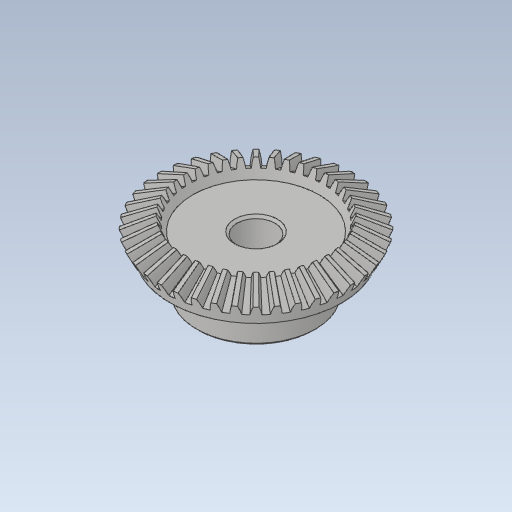
# Autodesk Inventor part: PB1-4020_On
Saved by Autodesk Inventor 2024 (Build 280153000, 153)
## iProperties
Created: 2023-09-03
Part Number: PB1-4020_On
Material: Generic
Catalog Web Link: www.cadenas.de
Description: Plastic Bevel Gears (PB)-R-
Vendor: KHK
Document SubType Name: Modeling
Designer: psAdmin
Manufacturer: KHK
Mass: 8.42838 g
Surface Area: 44.7487 cm^2
Volume: 8.42838 cm^3
Density: 1 g/cm^3
Appearance: PSOLRGB-175-175-175
Category: PARTsolutions
Company: KHK
PSOL_IDENT_0: {$CADENAS_DATA/23d-libs/khk/bevel_gears/pb_r.prj},185 {VTYP=3D},{NB=PB1-4020_On},{LINA=PB1-4020},{NN=
PSOL_IDENT_1: Plastic Bevel Gears (PB)-R},{DATE=06.10.2022 23:14:38},{GEOMDATE=20.03.2019 11:32:20},{VERSION=},{LI
PSOL_IDENT_2: NEID=340},{WBVAR=TOOTH},{WBNUMERIC=}  {NB=PB1-4020_On},{LINA=PB1-4020},{KT=DUMMY},{CN=PB1-4020},{M=1
PSOL_IDENT_3: .0},{Z=40},{A=8},{B=25},{C=40.0},{D=40.59},{E=22},{F=15.07},{G=12.59},{H=8.00},{I=12.0},{J=6},{K=26.
PSOL_IDENT_4: 58},{L=65.60},{S=B4},{PN=PB1-2040},{WMF=B4005.WMF},{X=0.5},{Y=0.5},{R=1.0},{H1=36.00},{VERS=5},{TOOT
PSOL_IDENT_5: H=On},{ANGLE=28.000}
NB: PB1-4020_On
NN: Plastic Bevel Gears (PB)-R
NBSYN: $CN._$TOOTH.
LINA: PB1-4020
CATALOG: KHK
CN: PB1-4020
M: 1
Z: 40
A: 8
B: 25
C: 40
D: 40.59
E: 22
F: 15.07
G: 12.59
H: 8
I: 12
J: 6
K: 26.58
L: 65.6
S: B4
PN: PB1-2040
WMF: B4005.WMF
X: 0.5
Y: 0.5
R: 1
H1: 36
VERS: 5
TOOTH: On
ANGLE: 28
SUPPLIER: KHK
ARTICLENO: PB1-4020_On
BOMINFO: PB1-4020
CREATOR: CADENAS GmbH
Title: PB1-4020
Author: Cadenas PARTsolutions
Autodesk Inventor part; units mm, degrees
sketch "Sketch_5" plane through (0, -14, 0) normal (0, 1, 0) x (1, 0, 0)
  arc A0 (-0.3975, 31.6288) -> (-0.999, 21.1842) centre (59.8613, 22.9187) ccw
  arc A1 (-0.999, 21.1842) -> (-2.3272, 21.0797) centre (0, 0) ccw
  arc A2 (-2.3272, 21.0797) -> (-4.5552, 31.3016) centre (-62.7095, 13.2721) ccw
  arc A3 (-4.5552, 31.3016) -> (-5.3404, 31.1772) centre (0, 0) ccw
  arc A4 (-5.3404, 31.1772) -> (-4.3007, 20.7671) centre (55.539, 32.0009) ccw
  arc A5 (-4.3007, 20.7671) -> (-5.5961, 20.4561) centre (0, 0) ccw
  arc A6 (-5.5961, 20.4561) -> (-9.3958, 30.2036) centre (-64.0137, 3.2988) ccw
  arc A7 (-9.3958, 30.2036) -> (-10.1519, 29.9579) centre (0, 0) ccw
  arc A8 (-10.1519, 29.9579) -> (-7.4964, 19.8387) centre (49.8492, 40.2951) ccw
  arc A9 (-7.4964, 19.8387) -> (-8.7273, 19.3288) centre (0, 0) ccw
  arc A10 (-8.7273, 19.3288) -> (-14.005, 28.3619) centre (-63.7416, -6.7558) ccw
  arc A11 (-14.005, 28.3619) -> (-14.7133, 28.001) centre (0, 0) ccw
  arc A12 (-14.7133, 28.001) -> (-10.5076, 18.4217) centre (42.9319, 47.5971) ccw
  arc A13 (-10.5076, 18.4217) -> (-11.6435, 17.7256) centre (0, 0) ccw
  arc A14 (-11.6435, 17.7256) -> (-18.2694, 25.8219) centre (-61.9, -16.644) ccw
  arc A15 (-18.2694, 25.8219) -> (-18.9125, 25.3546) centre (0, 0) ccw
  arc A16 (-18.9125, 25.3546) -> (-13.26, 16.5512) centre (34.9575, 53.7272) ccw
  arc A17 (-13.26, 16.5512) -> (-14.2731, 15.6859) centre (0, 0) ccw
  arc A18 (-14.2731, 15.6859) -> (-22.0839, 22.646) centre (-58.5343, -26.1224) ccw
  arc A19 (-22.0839, 22.646) -> (-22.646, 22.0839) centre (0, 0) ccw
  arc A20 (-22.646, 22.0839) -> (-15.6859, 14.2731) centre (26.1224, 58.5343) ccw
  arc A21 (-15.6859, 14.2731) -> (-16.5512, 13.26) centre (0, 0) ccw
  arc A22 (-16.5512, 13.26) -> (-25.3546, 18.9125) centre (-53.7272, -34.9575) ccw
  arc A23 (-25.3546, 18.9125) -> (-25.8219, 18.2694) centre (0, 0) ccw
  arc A24 (-25.8219, 18.2694) -> (-17.7256, 11.6435) centre (16.644, 61.9) ccw
  arc A25 (-17.7256, 11.6435) -> (-18.4217, 10.5076) centre (0, 0) ccw
  arc A26 (-18.4217, 10.5076) -> (-28.001, 14.7133) centre (-47.5971, -42.9319) ccw
  arc A27 (-28.001, 14.7133) -> (-28.3619, 14.005) centre (0, 0) ccw
  arc A28 (-28.3619, 14.005) -> (-19.3288, 8.7273) centre (6.7558, 63.7416) ccw
  arc A29 (-19.3288, 8.7273) -> (-19.8387, 7.4964) centre (0, 0) ccw
  arc A30 (-19.8387, 7.4964) -> (-29.9579, 10.1519) centre (-40.2951, -49.8492) ccw
  arc A31 (-29.9579, 10.1519) -> (-30.2036, 9.3958) centre (0, 0) ccw
  arc A32 (-30.2036, 9.3958) -> (-20.4561, 5.5961) centre (-3.2988, 64.0137) ccw
  arc A33 (-20.4561, 5.5961) -> (-20.7671, 4.3007) centre (0, 0) ccw
  arc A34 (-20.7671, 4.3007) -> (-31.1772, 5.3404) centre (-32.0009, -55.539) ccw
  arc A35 (-31.1772, 5.3404) -> (-31.3016, 4.5552) centre (0, 0) ccw
  arc A36 (-31.3016, 4.5552) -> (-21.0797, 2.3272) centre (-13.2721, 62.7095) ccw
  arc A37 (-21.0797, 2.3272) -> (-21.1842, 0.999) centre (0, 0) ccw
  arc A38 (-21.1842, 0.999) -> (-31.6288, 0.3975) centre (-22.9187, -59.8613) ccw
  arc A39 (-31.6288, 0.3975) -> (-31.6288, -0.3975) centre (0, 0) ccw
  arc A40 (-31.6288, -0.3975) -> (-21.1842, -0.999) centre (-22.9187, 59.8613) ccw
  arc A41 (-21.1842, -0.999) -> (-21.0797, -2.3272) centre (0, 0) ccw
  arc A42 (-21.0797, -2.3272) -> (-31.3016, -4.5552) centre (-13.2721, -62.7095) ccw
  arc A43 (-31.3016, -4.5552) -> (-31.1772, -5.3404) centre (0, 0) ccw
  arc A44 (-31.1772, -5.3404) -> (-20.7671, -4.3007) centre (-32.0009, 55.539) ccw
  arc A45 (-20.7671, -4.3007) -> (-20.4561, -5.5961) centre (0, 0) ccw
  arc A46 (-20.4561, -5.5961) -> (-30.2036, -9.3958) centre (-3.2988, -64.0137) ccw
  arc A47 (-30.2036, -9.3958) -> (-29.9579, -10.1519) centre (0, 0) ccw
  arc A48 (-29.9579, -10.1519) -> (-19.8387, -7.4964) centre (-40.2951, 49.8492) ccw
  arc A49 (-19.8387, -7.4964) -> (-19.3288, -8.7273) centre (0, 0) ccw
  arc A50 (-19.3288, -8.7273) -> (-28.3619, -14.005) centre (6.7558, -63.7416) ccw
  arc A51 (-28.3619, -14.005) -> (-28.001, -14.7133) centre (0, 0) ccw
  arc A52 (-28.001, -14.7133) -> (-18.4217, -10.5076) centre (-47.5971, 42.9319) ccw
  arc A53 (-18.4217, -10.5076) -> (-17.7256, -11.6435) centre (0, 0) ccw
  arc A54 (-17.7256, -11.6435) -> (-25.8219, -18.2694) centre (16.644, -61.9) ccw
  arc A55 (-25.8219, -18.2694) -> (-25.3546, -18.9125) centre (0, 0) ccw
  arc A56 (-25.3546, -18.9125) -> (-16.5512, -13.26) centre (-53.7272, 34.9575) ccw
  arc A57 (-16.5512, -13.26) -> (-15.6859, -14.2731) centre (0, 0) ccw
  arc A58 (-15.6859, -14.2731) -> (-22.646, -22.0839) centre (26.1224, -58.5343) ccw
  arc A59 (-22.646, -22.0839) -> (-22.0839, -22.646) centre (0, 0) ccw
  arc A60 (-22.0839, -22.646) -> (-14.2731, -15.6859) centre (-58.5343, 26.1224) ccw
  arc A61 (-14.2731, -15.6859) -> (-13.26, -16.5512) centre (0, 0) ccw
  arc A62 (-13.26, -16.5512) -> (-18.9125, -25.3546) centre (34.9575, -53.7272) ccw
  arc A63 (-18.9125, -25.3546) -> (-18.2694, -25.8219) centre (0, 0) ccw
  arc A64 (-18.2694, -25.8219) -> (-11.6435, -17.7256) centre (-61.9, 16.644) ccw
  arc A65 (-11.6435, -17.7256) -> (-10.5076, -18.4217) centre (0, 0) ccw
  arc A66 (-10.5076, -18.4217) -> (-14.7133, -28.001) centre (42.9319, -47.5971) ccw
  arc A67 (-14.7133, -28.001) -> (-14.005, -28.3619) centre (0, 0) ccw
  arc A68 (-14.005, -28.3619) -> (-8.7273, -19.3288) centre (-63.7416, 6.7558) ccw
  arc A69 (-8.7273, -19.3288) -> (-7.4964, -19.8387) centre (0, 0) ccw
  arc A70 (-7.4964, -19.8387) -> (-10.1519, -29.9579) centre (49.8492, -40.2951) ccw
  arc A71 (-10.1519, -29.9579) -> (-9.3958, -30.2036) centre (0, 0) ccw
  arc A72 (-9.3958, -30.2036) -> (-5.5961, -20.4561) centre (-64.0137, -3.2988) ccw
  arc A73 (-5.5961, -20.4561) -> (-4.3007, -20.7671) centre (0, 0) ccw
  arc A74 (-4.3007, -20.7671) -> (-5.3404, -31.1772) centre (55.539, -32.0009) ccw
  arc A75 (-5.3404, -31.1772) -> (-4.5552, -31.3016) centre (0, 0) ccw
  arc A76 (-4.5552, -31.3016) -> (-2.3272, -21.0797) centre (-62.7095, -13.2721) ccw
  arc A77 (-2.3272, -21.0797) -> (-0.999, -21.1842) centre (0, 0) ccw
  arc A78 (-0.999, -21.1842) -> (-0.3975, -31.6288) centre (59.8613, -22.9187) ccw
  arc A79 (-0.3975, -31.6288) -> (0.3975, -31.6288) centre (0, 0) ccw
  arc A80 (0.3975, -31.6288) -> (0.999, -21.1842) centre (-59.8613, -22.9187) ccw
  arc A81 (0.999, -21.1842) -> (2.3272, -21.0797) centre (0, 0) ccw
  arc A82 (2.3272, -21.0797) -> (4.5552, -31.3016) centre (62.7095, -13.2721) ccw
  arc A83 (4.5552, -31.3016) -> (5.3404, -31.1772) centre (0, 0) ccw
  arc A84 (5.3404, -31.1772) -> (4.3007, -20.7671) centre (-55.539, -32.0009) ccw
  arc A85 (4.3007, -20.7671) -> (5.5961, -20.4561) centre (0, 0) ccw
  arc A86 (5.5961, -20.4561) -> (9.3958, -30.2036) centre (64.0137, -3.2988) ccw
  arc A87 (9.3958, -30.2036) -> (10.1519, -29.9579) centre (0, 0) ccw
  arc A88 (10.1519, -29.9579) -> (7.4964, -19.8387) centre (-49.8492, -40.2951) ccw
  arc A89 (7.4964, -19.8387) -> (8.7273, -19.3288) centre (0, 0) ccw
  arc A90 (8.7273, -19.3288) -> (14.005, -28.3619) centre (63.7416, 6.7558) ccw
  arc A91 (14.005, -28.3619) -> (14.7133, -28.001) centre (0, 0) ccw
  arc A92 (14.7133, -28.001) -> (10.5076, -18.4217) centre (-42.9319, -47.5971) ccw
  arc A93 (10.5076, -18.4217) -> (11.6435, -17.7256) centre (0, 0) ccw
  arc A94 (11.6435, -17.7256) -> (18.2694, -25.8219) centre (61.9, 16.644) ccw
  arc A95 (18.2694, -25.8219) -> (18.9125, -25.3546) centre (0, 0) ccw
  arc A96 (18.9125, -25.3546) -> (13.26, -16.5512) centre (-34.9575, -53.7272) ccw
  arc A97 (13.26, -16.5512) -> (14.2731, -15.6859) centre (0, 0) ccw
  arc A98 (14.2731, -15.6859) -> (22.0839, -22.646) centre (58.5343, 26.1224) ccw
  arc A99 (22.0839, -22.646) -> (22.646, -22.0839) centre (0, 0) ccw
  arc A100 (22.646, -22.0839) -> (15.6859, -14.2731) centre (-26.1224, -58.5343) ccw
  arc A101 (15.6859, -14.2731) -> (16.5512, -13.26) centre (0, 0) ccw
  arc A102 (16.5512, -13.26) -> (25.3546, -18.9125) centre (53.7272, 34.9575) ccw
  arc A103 (25.3546, -18.9125) -> (25.8219, -18.2694) centre (0, 0) ccw
  arc A104 (25.8219, -18.2694) -> (17.7256, -11.6435) centre (-16.644, -61.9) ccw
  arc A105 (17.7256, -11.6435) -> (18.4217, -10.5076) centre (0, 0) ccw
  arc A106 (18.4217, -10.5076) -> (28.001, -14.7133) centre (47.5971, 42.9319) ccw
  arc A107 (28.001, -14.7133) -> (28.3619, -14.005) centre (0, 0) ccw
  arc A108 (28.3619, -14.005) -> (19.3288, -8.7273) centre (-6.7558, -63.7416) ccw
  arc A109 (19.3288, -8.7273) -> (19.8387, -7.4964) centre (0, 0) ccw
  arc A110 (19.8387, -7.4964) -> (29.9579, -10.1519) centre (40.2951, 49.8492) ccw
  arc A111 (29.9579, -10.1519) -> (30.2036, -9.3958) centre (0, 0) ccw
  arc A112 (30.2036, -9.3958) -> (20.4561, -5.5961) centre (3.2988, -64.0137) ccw
  arc A113 (20.4561, -5.5961) -> (20.7671, -4.3007) centre (0, 0) ccw
  arc A114 (20.7671, -4.3007) -> (31.1772, -5.3404) centre (32.0009, 55.539) ccw
  arc A115 (31.1772, -5.3404) -> (31.3016, -4.5552) centre (0, 0) ccw
  arc A116 (31.3016, -4.5552) -> (21.0797, -2.3272) centre (13.2721, -62.7095) ccw
  arc A117 (21.0797, -2.3272) -> (21.1842, -0.999) centre (0, 0) ccw
  arc A118 (21.1842, -0.999) -> (31.6288, -0.3975) centre (22.9187, 59.8613) ccw
  arc A119 (31.6288, -0.3975) -> (31.6288, 0.3975) centre (0, 0) ccw
  arc A120 (31.6288, 0.3975) -> (21.1842, 0.999) centre (22.9187, -59.8613) ccw
  arc A121 (21.1842, 0.999) -> (21.0797, 2.3272) centre (0, 0) ccw
  arc A122 (21.0797, 2.3272) -> (31.3016, 4.5552) centre (13.2721, 62.7095) ccw
  arc A123 (31.3016, 4.5552) -> (31.1772, 5.3404) centre (0, 0) ccw
  arc A124 (31.1772, 5.3404) -> (20.7671, 4.3007) centre (32.0009, -55.539) ccw
  arc A125 (20.7671, 4.3007) -> (20.4561, 5.5961) centre (0, 0) ccw
  arc A126 (20.4561, 5.5961) -> (30.2036, 9.3958) centre (3.2988, 64.0137) ccw
  arc A127 (30.2036, 9.3958) -> (29.9579, 10.1519) centre (0, 0) ccw
  arc A128 (29.9579, 10.1519) -> (19.8387, 7.4964) centre (40.2951, -49.8492) ccw
  arc A129 (19.8387, 7.4964) -> (19.3288, 8.7273) centre (0, 0) ccw
  arc A130 (19.3288, 8.7273) -> (28.3619, 14.005) centre (-6.7558, 63.7416) ccw
  arc A131 (28.3619, 14.005) -> (28.001, 14.7133) centre (0, 0) ccw
  arc A132 (28.001, 14.7133) -> (18.4217, 10.5076) centre (47.5971, -42.9319) ccw
  arc A133 (18.4217, 10.5076) -> (17.7256, 11.6435) centre (0, 0) ccw
  arc A134 (17.7256, 11.6435) -> (25.8219, 18.2694) centre (-16.644, 61.9) ccw
  arc A135 (25.8219, 18.2694) -> (25.3546, 18.9125) centre (0, 0) ccw
  arc A136 (25.3546, 18.9125) -> (16.5512, 13.26) centre (53.7272, -34.9575) ccw
  arc A137 (16.5512, 13.26) -> (15.6859, 14.2731) centre (0, 0) ccw
  arc A138 (15.6859, 14.2731) -> (22.646, 22.0839) centre (-26.1224, 58.5343) ccw
  arc A139 (22.646, 22.0839) -> (22.0839, 22.646) centre (0, 0) ccw
  arc A140 (22.0839, 22.646) -> (14.2731, 15.6859) centre (58.5343, -26.1224) ccw
  arc A141 (14.2731, 15.6859) -> (13.26, 16.5512) centre (0, 0) ccw
  arc A142 (13.26, 16.5512) -> (18.9125, 25.3546) centre (-34.9575, 53.7272) ccw
  arc A143 (18.9125, 25.3546) -> (18.2694, 25.8219) centre (0, 0) ccw
  arc A144 (18.2694, 25.8219) -> (11.6435, 17.7256) centre (61.9, -16.644) ccw
  arc A145 (11.6435, 17.7256) -> (10.5076, 18.4217) centre (0, 0) ccw
  arc A146 (10.5076, 18.4217) -> (14.7133, 28.001) centre (-42.9319, 47.5971) ccw
  arc A147 (14.7133, 28.001) -> (14.005, 28.3619) centre (0, 0) ccw
  arc A148 (14.005, 28.3619) -> (8.7273, 19.3288) centre (63.7416, -6.7558) ccw
  arc A149 (8.7273, 19.3288) -> (7.4964, 19.8387) centre (0, 0) ccw
  arc A150 (7.4964, 19.8387) -> (10.1519, 29.9579) centre (-49.8492, 40.2951) ccw
  arc A151 (10.1519, 29.9579) -> (9.3958, 30.2036) centre (0, 0) ccw
  arc A152 (9.3958, 30.2036) -> (5.5961, 20.4561) centre (64.0137, 3.2988) ccw
  arc A153 (5.5961, 20.4561) -> (4.3007, 20.7671) centre (0, 0) ccw
  arc A154 (4.3007, 20.7671) -> (5.3404, 31.1772) centre (-55.539, 32.0009) ccw
  arc A155 (5.3404, 31.1772) -> (4.5552, 31.3016) centre (0, 0) ccw
  arc A156 (4.5552, 31.3016) -> (2.3272, 21.0797) centre (62.7095, 13.2721) ccw
  arc A157 (2.3272, 21.0797) -> (0.999, 21.1842) centre (0, 0) ccw
  arc A158 (0.999, 21.1842) -> (0.3975, 31.6288) centre (-59.8613, 22.9187) ccw
  arc A159 (0.3975, 31.6288) -> (-0.3975, 31.6288) centre (0, 0) ccw
  constraints: 320 point on circle, 160 centre point
sketch "Sketch_6" plane through (0, -6.93, 0) normal (0, 1, 0) x (1, 0, 0)
  arc A0 (-0.2948, 15.6369) -> (-0.61, 9.6964) centre (39.9716, 10.5213) ccw
  arc A1 (-0.61, 9.6964) -> (-0.9143, 9.6725) centre (0, 0) ccw
  arc A2 (-0.9143, 9.6725) -> (-2.155, 15.4905) centre (-41.1254, 4.1389) ccw
  arc A3 (-2.155, 15.4905) -> (-2.7373, 15.3983) centre (0, 0) ccw
  arc A4 (-2.7373, 15.3983) -> (-2.1194, 9.4816) centre (37.8336, 16.6447) ccw
  arc A5 (-2.1194, 9.4816) -> (-2.4162, 9.4104) centre (0, 0) ccw
  arc A6 (-2.4162, 9.4104) -> (-4.5517, 14.9627) centre (-41.2665, -2.3455) ccw
  arc A7 (-4.5517, 14.9627) -> (-5.1124, 14.7805) centre (0, 0) ccw
  arc A8 (-5.1124, 14.7805) -> (-3.5766, 9.0334) centre (34.764, 22.3583) ccw
  arc A9 (-3.5766, 9.0334) -> (-3.8585, 8.9166) centre (0, 0) ccw
  arc A10 (-3.8585, 8.9166) -> (-6.8363, 14.0664) centre (-40.3915, -8.7721) ccw
  arc A11 (-6.8363, 14.0664) -> (-7.3617, 13.7987) centre (0, 0) ccw
  arc A12 (-7.3617, 13.7987) -> (-4.9457, 8.3626) centre (30.8383, 27.5213) ccw
  arc A13 (-4.9457, 8.3626) -> (-5.2059, 8.2032) centre (0, 0) ccw
  arc A14 (-5.2059, 8.2032) -> (-8.9526, 12.8238) centre (-38.522, -14.9828) ccw
  arc A15 (-8.9526, 12.8238) -> (-9.4296, 12.4772) centre (0, 0) ccw
  arc A16 (-9.4296, 12.4772) -> (-6.193, 7.486) centre (26.1534, 32.0066) ccw
  arc A17 (-6.193, 7.486) -> (-6.4251, 7.2878) centre (0, 0) ccw
  arc A18 (-6.4251, 7.2878) -> (-10.8485, 11.2654) centre (-35.7039, -20.8245) ccw
  arc A19 (-10.8485, 11.2654) -> (-11.2654, 10.8485) centre (0, 0) ccw
  arc A20 (-11.2654, 10.8485) -> (-7.2878, 6.4251) centre (20.8245, 35.7039) ccw
  arc A21 (-7.2878, 6.4251) -> (-7.486, 6.193) centre (0, 0) ccw
  arc A22 (-7.486, 6.193) -> (-12.4772, 9.4296) centre (-32.0066, -26.1534) ccw
  arc A23 (-12.4772, 9.4296) -> (-12.8238, 8.9526) centre (0, 0) ccw
  arc A24 (-12.8238, 8.9526) -> (-8.2032, 5.2059) centre (14.9828, 38.522) ccw
  arc A25 (-8.2032, 5.2059) -> (-8.3626, 4.9457) centre (0, 0) ccw
  arc A26 (-8.3626, 4.9457) -> (-13.7987, 7.3617) centre (-27.5213, -30.8383) ccw
  arc A27 (-13.7987, 7.3617) -> (-14.0664, 6.8363) centre (0, 0) ccw
  arc A28 (-14.0664, 6.8363) -> (-8.9166, 3.8585) centre (8.7721, 40.3915) ccw
  arc A29 (-8.9166, 3.8585) -> (-9.0334, 3.5766) centre (0, 0) ccw
  arc A30 (-9.0334, 3.5766) -> (-14.7805, 5.1124) centre (-22.3583, -34.764) ccw
  arc A31 (-14.7805, 5.1124) -> (-14.9627, 4.5517) centre (0, 0) ccw
  arc A32 (-14.9627, 4.5517) -> (-9.4104, 2.4162) centre (2.3455, 41.2665) ccw
  arc A33 (-9.4104, 2.4162) -> (-9.4816, 2.1194) centre (0, 0) ccw
  arc A34 (-9.4816, 2.1194) -> (-15.3983, 2.7373) centre (-16.6447, -37.8336) ccw
  arc A35 (-15.3983, 2.7373) -> (-15.4905, 2.155) centre (0, 0) ccw
  arc A36 (-15.4905, 2.155) -> (-9.6725, 0.9143) centre (-4.1389, 41.1254) ccw
  arc A37 (-9.6725, 0.9143) -> (-9.6964, 0.61) centre (0, 0) ccw
  arc A38 (-9.6964, 0.61) -> (-15.6369, 0.2948) centre (-10.5213, -39.9716) ccw
  arc A39 (-15.6369, 0.2948) -> (-15.6369, -0.2948) centre (0, 0) ccw
  arc A40 (-15.6369, -0.2948) -> (-9.6964, -0.61) centre (-10.5213, 39.9716) ccw
  arc A41 (-9.6964, -0.61) -> (-9.6725, -0.9143) centre (0, 0) ccw
  arc A42 (-9.6725, -0.9143) -> (-15.4905, -2.155) centre (-4.1389, -41.1254) ccw
  arc A43 (-15.4905, -2.155) -> (-15.3983, -2.7373) centre (0, 0) ccw
  arc A44 (-15.3983, -2.7373) -> (-9.4816, -2.1194) centre (-16.6447, 37.8336) ccw
  arc A45 (-9.4816, -2.1194) -> (-9.4104, -2.4162) centre (0, 0) ccw
  arc A46 (-9.4104, -2.4162) -> (-14.9627, -4.5517) centre (2.3455, -41.2665) ccw
  arc A47 (-14.9627, -4.5517) -> (-14.7805, -5.1124) centre (0, 0) ccw
  arc A48 (-14.7805, -5.1124) -> (-9.0334, -3.5766) centre (-22.3583, 34.764) ccw
  arc A49 (-9.0334, -3.5766) -> (-8.9166, -3.8585) centre (0, 0) ccw
  arc A50 (-8.9166, -3.8585) -> (-14.0664, -6.8363) centre (8.7721, -40.3915) ccw
  arc A51 (-14.0664, -6.8363) -> (-13.7987, -7.3617) centre (0, 0) ccw
  arc A52 (-13.7987, -7.3617) -> (-8.3626, -4.9457) centre (-27.5213, 30.8383) ccw
  arc A53 (-8.3626, -4.9457) -> (-8.2032, -5.2059) centre (0, 0) ccw
  arc A54 (-8.2032, -5.2059) -> (-12.8238, -8.9526) centre (14.9828, -38.522) ccw
  arc A55 (-12.8238, -8.9526) -> (-12.4772, -9.4296) centre (0, 0) ccw
  arc A56 (-12.4772, -9.4296) -> (-7.486, -6.193) centre (-32.0066, 26.1534) ccw
  arc A57 (-7.486, -6.193) -> (-7.2878, -6.4251) centre (0, 0) ccw
  arc A58 (-7.2878, -6.4251) -> (-11.2654, -10.8485) centre (20.8245, -35.7039) ccw
  arc A59 (-11.2654, -10.8485) -> (-10.8485, -11.2654) centre (0, 0) ccw
  arc A60 (-10.8485, -11.2654) -> (-6.4251, -7.2878) centre (-35.7039, 20.8245) ccw
  arc A61 (-6.4251, -7.2878) -> (-6.193, -7.486) centre (0, 0) ccw
  arc A62 (-6.193, -7.486) -> (-9.4296, -12.4772) centre (26.1534, -32.0066) ccw
  arc A63 (-9.4296, -12.4772) -> (-8.9526, -12.8238) centre (0, 0) ccw
  arc A64 (-8.9526, -12.8238) -> (-5.2059, -8.2032) centre (-38.522, 14.9828) ccw
  arc A65 (-5.2059, -8.2032) -> (-4.9457, -8.3626) centre (0, 0) ccw
  arc A66 (-4.9457, -8.3626) -> (-7.3617, -13.7987) centre (30.8383, -27.5213) ccw
  arc A67 (-7.3617, -13.7987) -> (-6.8363, -14.0664) centre (0, 0) ccw
  arc A68 (-6.8363, -14.0664) -> (-3.8585, -8.9166) centre (-40.3915, 8.7721) ccw
  arc A69 (-3.8585, -8.9166) -> (-3.5766, -9.0334) centre (0, 0) ccw
  arc A70 (-3.5766, -9.0334) -> (-5.1124, -14.7805) centre (34.764, -22.3583) ccw
  arc A71 (-5.1124, -14.7805) -> (-4.5517, -14.9627) centre (0, 0) ccw
  arc A72 (-4.5517, -14.9627) -> (-2.4162, -9.4104) centre (-41.2665, 2.3455) ccw
  arc A73 (-2.4162, -9.4104) -> (-2.1194, -9.4816) centre (0, 0) ccw
  arc A74 (-2.1194, -9.4816) -> (-2.7373, -15.3983) centre (37.8336, -16.6447) ccw
  arc A75 (-2.7373, -15.3983) -> (-2.155, -15.4905) centre (0, 0) ccw
  arc A76 (-2.155, -15.4905) -> (-0.9143, -9.6725) centre (-41.1254, -4.1389) ccw
  arc A77 (-0.9143, -9.6725) -> (-0.61, -9.6964) centre (0, 0) ccw
  arc A78 (-0.61, -9.6964) -> (-0.2948, -15.6369) centre (39.9716, -10.5213) ccw
  arc A79 (-0.2948, -15.6369) -> (0.2948, -15.6369) centre (0, 0) ccw
  arc A80 (0.2948, -15.6369) -> (0.61, -9.6964) centre (-39.9716, -10.5213) ccw
  arc A81 (0.61, -9.6964) -> (0.9143, -9.6725) centre (0, 0) ccw
  arc A82 (0.9143, -9.6725) -> (2.155, -15.4905) centre (41.1254, -4.1389) ccw
  arc A83 (2.155, -15.4905) -> (2.7373, -15.3983) centre (0, 0) ccw
  arc A84 (2.7373, -15.3983) -> (2.1194, -9.4816) centre (-37.8336, -16.6447) ccw
  arc A85 (2.1194, -9.4816) -> (2.4162, -9.4104) centre (0, 0) ccw
  arc A86 (2.4162, -9.4104) -> (4.5517, -14.9627) centre (41.2665, 2.3455) ccw
  arc A87 (4.5517, -14.9627) -> (5.1124, -14.7805) centre (0, 0) ccw
  arc A88 (5.1124, -14.7805) -> (3.5766, -9.0334) centre (-34.764, -22.3583) ccw
  arc A89 (3.5766, -9.0334) -> (3.8585, -8.9166) centre (0, 0) ccw
  arc A90 (3.8585, -8.9166) -> (6.8363, -14.0664) centre (40.3915, 8.7721) ccw
  arc A91 (6.8363, -14.0664) -> (7.3617, -13.7987) centre (0, 0) ccw
  arc A92 (7.3617, -13.7987) -> (4.9457, -8.3626) centre (-30.8383, -27.5213) ccw
  arc A93 (4.9457, -8.3626) -> (5.2059, -8.2032) centre (0, 0) ccw
  arc A94 (5.2059, -8.2032) -> (8.9526, -12.8238) centre (38.522, 14.9828) ccw
  arc A95 (8.9526, -12.8238) -> (9.4296, -12.4772) centre (0, 0) ccw
  arc A96 (9.4296, -12.4772) -> (6.193, -7.486) centre (-26.1534, -32.0066) ccw
  arc A97 (6.193, -7.486) -> (6.4251, -7.2878) centre (0, 0) ccw
  arc A98 (6.4251, -7.2878) -> (10.8485, -11.2654) centre (35.7039, 20.8245) ccw
  arc A99 (10.8485, -11.2654) -> (11.2654, -10.8485) centre (0, 0) ccw
  arc A100 (11.2654, -10.8485) -> (7.2878, -6.4251) centre (-20.8245, -35.7039) ccw
  arc A101 (7.2878, -6.4251) -> (7.486, -6.193) centre (0, 0) ccw
  arc A102 (7.486, -6.193) -> (12.4772, -9.4296) centre (32.0066, 26.1534) ccw
  arc A103 (12.4772, -9.4296) -> (12.8238, -8.9526) centre (0, 0) ccw
  arc A104 (12.8238, -8.9526) -> (8.2032, -5.2059) centre (-14.9828, -38.522) ccw
  arc A105 (8.2032, -5.2059) -> (8.3626, -4.9457) centre (0, 0) ccw
  arc A106 (8.3626, -4.9457) -> (13.7987, -7.3617) centre (27.5213, 30.8383) ccw
  arc A107 (13.7987, -7.3617) -> (14.0664, -6.8363) centre (0, 0) ccw
  arc A108 (14.0664, -6.8363) -> (8.9166, -3.8585) centre (-8.7721, -40.3915) ccw
  arc A109 (8.9166, -3.8585) -> (9.0334, -3.5766) centre (0, 0) ccw
  arc A110 (9.0334, -3.5766) -> (14.7805, -5.1124) centre (22.3583, 34.764) ccw
  arc A111 (14.7805, -5.1124) -> (14.9627, -4.5517) centre (0, 0) ccw
  arc A112 (14.9627, -4.5517) -> (9.4104, -2.4162) centre (-2.3455, -41.2665) ccw
  arc A113 (9.4104, -2.4162) -> (9.4816, -2.1194) centre (0, 0) ccw
  arc A114 (9.4816, -2.1194) -> (15.3983, -2.7373) centre (16.6447, 37.8336) ccw
  arc A115 (15.3983, -2.7373) -> (15.4905, -2.155) centre (0, 0) ccw
  arc A116 (15.4905, -2.155) -> (9.6725, -0.9143) centre (4.1389, -41.1254) ccw
  arc A117 (9.6725, -0.9143) -> (9.6964, -0.61) centre (0, 0) ccw
  arc A118 (9.6964, -0.61) -> (15.6369, -0.2948) centre (10.5213, 39.9716) ccw
  arc A119 (15.6369, -0.2948) -> (15.6369, 0.2948) centre (0, 0) ccw
  arc A120 (15.6369, 0.2948) -> (9.6964, 0.61) centre (10.5213, -39.9716) ccw
  arc A121 (9.6964, 0.61) -> (9.6725, 0.9143) centre (0, 0) ccw
  arc A122 (9.6725, 0.9143) -> (15.4905, 2.155) centre (4.1389, 41.1254) ccw
  arc A123 (15.4905, 2.155) -> (15.3983, 2.7373) centre (0, 0) ccw
  arc A124 (15.3983, 2.7373) -> (9.4816, 2.1194) centre (16.6447, -37.8336) ccw
  arc A125 (9.4816, 2.1194) -> (9.4104, 2.4162) centre (0, 0) ccw
  arc A126 (9.4104, 2.4162) -> (14.9627, 4.5517) centre (-2.3455, 41.2665) ccw
  arc A127 (14.9627, 4.5517) -> (14.7805, 5.1124) centre (0, 0) ccw
  arc A128 (14.7805, 5.1124) -> (9.0334, 3.5766) centre (22.3583, -34.764) ccw
  arc A129 (9.0334, 3.5766) -> (8.9166, 3.8585) centre (0, 0) ccw
  arc A130 (8.9166, 3.8585) -> (14.0664, 6.8363) centre (-8.7721, 40.3915) ccw
  arc A131 (14.0664, 6.8363) -> (13.7987, 7.3617) centre (0, 0) ccw
  arc A132 (13.7987, 7.3617) -> (8.3626, 4.9457) centre (27.5213, -30.8383) ccw
  arc A133 (8.3626, 4.9457) -> (8.2032, 5.2059) centre (0, 0) ccw
  arc A134 (8.2032, 5.2059) -> (12.8238, 8.9526) centre (-14.9828, 38.522) ccw
  arc A135 (12.8238, 8.9526) -> (12.4772, 9.4296) centre (0, 0) ccw
  arc A136 (12.4772, 9.4296) -> (7.486, 6.193) centre (32.0066, -26.1534) ccw
  arc A137 (7.486, 6.193) -> (7.2878, 6.4251) centre (0, 0) ccw
  arc A138 (7.2878, 6.4251) -> (11.2654, 10.8485) centre (-20.8245, 35.7039) ccw
  arc A139 (11.2654, 10.8485) -> (10.8485, 11.2654) centre (0, 0) ccw
  arc A140 (10.8485, 11.2654) -> (6.4251, 7.2878) centre (35.7039, -20.8245) ccw
  arc A141 (6.4251, 7.2878) -> (6.193, 7.486) centre (0, 0) ccw
  arc A142 (6.193, 7.486) -> (9.4296, 12.4772) centre (-26.1534, 32.0066) ccw
  arc A143 (9.4296, 12.4772) -> (8.9526, 12.8238) centre (0, 0) ccw
  arc A144 (8.9526, 12.8238) -> (5.2059, 8.2032) centre (38.522, -14.9828) ccw
  arc A145 (5.2059, 8.2032) -> (4.9457, 8.3626) centre (0, 0) ccw
  arc A146 (4.9457, 8.3626) -> (7.3617, 13.7987) centre (-30.8383, 27.5213) ccw
  arc A147 (7.3617, 13.7987) -> (6.8363, 14.0664) centre (0, 0) ccw
  arc A148 (6.8363, 14.0664) -> (3.8585, 8.9166) centre (40.3915, -8.7721) ccw
  arc A149 (3.8585, 8.9166) -> (3.5766, 9.0334) centre (0, 0) ccw
  arc A150 (3.5766, 9.0334) -> (5.1124, 14.7805) centre (-34.764, 22.3583) ccw
  arc A151 (5.1124, 14.7805) -> (4.5517, 14.9627) centre (0, 0) ccw
  arc A152 (4.5517, 14.9627) -> (2.4162, 9.4104) centre (41.2665, -2.3455) ccw
  arc A153 (2.4162, 9.4104) -> (2.1194, 9.4816) centre (0, 0) ccw
  arc A154 (2.1194, 9.4816) -> (2.7373, 15.3983) centre (-37.8336, 16.6447) ccw
  arc A155 (2.7373, 15.3983) -> (2.155, 15.4905) centre (0, 0) ccw
  arc A156 (2.155, 15.4905) -> (0.9143, 9.6725) centre (41.1254, 4.1389) ccw
  arc A157 (0.9143, 9.6725) -> (0.61, 9.6964) centre (0, 0) ccw
  arc A158 (0.61, 9.6964) -> (0.2948, 15.6369) centre (-39.9716, 10.5213) ccw
  arc A159 (0.2948, 15.6369) -> (-0.2948, 15.6369) centre (0, 0) ccw
  constraints: 320 point on circle, 160 centre point
loft "Loft1" add profiles "Sketch_5", "Sketch_6"
sketch "Sketch_7" plane through (0, 0, 0) normal (0, 0, 1) x (1, 0, 0)
  line L0 (0, -6.93) -> (0, -22)
  line L1 (0, -22) -> (-12, -22)
  line L2 (-12, -22) -> (-12.5, -21.5)
  line L3 (-12.5, -21.5) -> (-12.5, -15)
  arc A0 (-12.5, -15) -> (-13.5, -14) centre (-13.5, -15) ccw
  line L4 (-13.5, -14) -> (-18, -14)
  line L5 (-18, -14) -> (-19.2023, -11.5954)
  line L6 (-19.2023, -11.5954) -> (-14.0729, -8.4398)
  line L7 (-14.0729, -8.4398) -> (-13.2929, -10)
  line L8 (-13.2929, -10) -> (0, -10)
  line L9 (0, -10) -> (0, -22)
  constraints: 20 end point, 2 point on circle, 1 centre point
revolve "Revolution1" add sketch "Sketch_7" angle 360 about axis through (0, -6.93, 0) along (0, 1, 0)
sketch "Sketch_8" plane through (0, 0, 0) normal (0, 0, 1) x (1, 0, 0)
  line L0 (0, 0) -> (0, -22)
  line L1 (0, -22) -> (-4.5, -22)
  line L2 (-4.5, -22) -> (-4, -21.5)
  line L3 (-4, -21.5) -> (-4, -10.5)
  line L4 (-4, -10.5) -> (-4.5, -10)
  line L5 (-4.5, -10) -> (-13.2929, -10)
  line L6 (-13.2929, -10) -> (-14.8279, -6.93)
  line L7 (-14.8279, -6.93) -> (-20.295, -9.41)
  line L8 (-20.295, -9.41) -> (-18, -14)
  line L9 (-18, -14) -> (-40.59, -14)
  line L10 (-40.59, -14) -> (-40.59, 0)
  line L11 (-40.59, 0) -> (0, 0)
  line L12 (0, 0) -> (0, -22)
  constraints: 26 end point
revolve "Revolution2" cut sketch "Sketch_8" angle 360 about axis through (0, 0, 0) along (0, 1, 0)
ref_plane "IP2_XY" through (0, 0, 0) normal (0, 0, 1) x (1, 0, 0)
ref_plane "IP2_YZ" through (0, 0, 0) normal (1, 0, 0) x (0, 1, 0)
ref_plane "IP2_ZX" through (0, 0, 0) normal (0, 1, 0) x (0, 0, 1)
ref_plane "dummy_XY" through (0, 0, 0) normal (0, 1, 0) x (1, 0, 0)
ref_plane "dummy_YZ" through (0, 0, 0) normal (1, 0, 0) x (0, 0, -1)
ref_plane "dummy_ZX" through (0, 0, 0) normal (0, 0, -1) x (0, 1, 0)
ref_plane "r_XY" through (0, 0, 0) normal (0, 1, 0) x (1, 0, 0)
ref_plane "r_YZ" through (0, 0, 0) normal (1, 0, 0) x (0, 0, -1)
ref_plane "r_ZX" through (0, 0, 0) normal (0, 0, -1) x (0, 1, 0)
body "Solid1"
